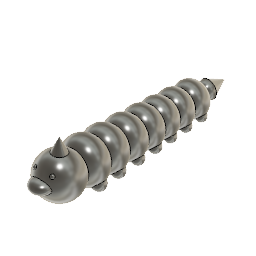
imomushi (Autodesk Fusion 360 design; units mm, degrees)
Autodesk Fusion 360 part; units mm, degrees
note: some values were not read from the file. Set by a fixed rule: which sketch regions a step uses.
sketch "スケッチ1" plane through (0, 0, 0) normal (0, 1, 0) x (1, 0, 0)
  line L0 (0, 0) -> (0, -20)
  line L1 (0, 0) -> (10, 0)
  line L2 (10, 0) -> (0, -20)
  arc A0 (10, 0) -> (0, 10) centre (0, 0) ccw
  line L3 (0, 0) -> (0, 10)
  ellipse E0 centre (0, 0) end of major axis (0, -7.5) minor radius 12.5
  line L4 (0, 7.5) -> (0, -7.5)
  line L5 (-12.5, 0) -> (12.5, 0)
  ellipse E1 centre (0, 0) end of major axis (0, -20) minor radius 25
  line L6 (0, 20) -> (0, -20)
  line L7 (-25, 0) -> (25, 0)
  circle A1 centre (0, 0) radius 7.5
  line L8 (0, -20) -> (0, 20)
  dimension "d1" = 20
  dimension "d2" = 10
  dimension "d8" = 15
  dimension "d9" = 25
  constraint coincident L0.start L1.start
  constraint vertical L0
  constraint perpendicular L0 L1
  constraint perpendicular L1 L3
  constraint perpendicular L1 L4
  constraint coincident E0 L4.start
  constraint coincident E0 L4.end
  constraint coincident E0 L5.start
  constraint coincident E0 L5.end
  constraint concentric A0 E1
  constraint parallel L0 L6
  constraint coincident E1 L6.start
  constraint coincident E1 L7.start
  constraint coincident E1 L7.end
  constraint coincident L4.end A1
  constraint parallel L6 L8
  measures "d1" distance of L0.start L0.end
  measures "d2" distance of L0.start L1.end
  measures "d8" distance of E0
revolve "回転1" add sketch "スケッチ1" angle 360 about axis through (0, 0, 1.75) along (0, 0, 1) contours L0 L1 L4 L5 L6 L7 A1 L8 | L0 L2 E0 L6 L8 | L1 L2 E0 L5 L7 A1 makes body 1
revolve "回転2" add sketch "スケッチ1" angle 360 about axis through (0, 0, 1.75) along (0, 0, 1) separate body contours L0 L1 L4 L5 L6 L7 A1 L8 | L1 L3 L4 L5 L6 L7 A1 L8 | L0 L2 E0 L6 L8 | L1 L2 E0 L5 L7 A1 | L1 A0 E0 L5 L7 A1 | A0 L3 E0 L6 L8 makes body 2
move_body "移動1" bodies 1 to x (1, 0, 0) y (0, 1, 0) z (0, 0, 1) at (0, 0, 20)
sphere "球プリミティブ1" add diameter 50 placed x (1, 0, 0) y (0, 0, -1) z (0, 1, 0) at (0, 0, 0) separate body makes body 3
sphere "球プリミティブ2" add diameter 5 placed x (1, 0, 0) y (0, 0, -1) z (0, 1, 0) at (0, 0, 0) separate body makes body 4
move_body "移動2" bodies 4 to x (1, 0, 0) y (0, 1, 0) z (0, 0, 1) at (10.0469, -18.3305, 12.2249)
mirror "ミラー1" about plane through (0, 0, 0) normal (1, 0, 0) of bodies 4 makes body 5
revolve "回転3" add sketch "スケッチ1" angle 360 about axis through (0, 0, 1.75) along (0, 0, 1) separate body contours L0 L1 L4 L5 L6 L7 A1 L8 | L1 L3 L4 L5 L6 L7 A1 L8 | L1 L2 E0 L5 L7 A1 | L1 A0 E0 L5 L7 A1 | L2 E0 L5 L7 | A0 E0 L5 L7 makes body 6
move_body "移動3" bodies 6 to x (1, 0, 0) y (0, 1, 0) z (0, 0, 1) at (0, -21.5417, 0)
revolve "回転4" add sketch "スケッチ1" angle 360 about axis through (0, 0, 1.75) along (0, 0, 1) separate body contours L0 L1 L4 L5 L6 L7 A1 L8 | L1 L3 L4 L5 L6 L7 A1 L8 | L0 L2 E0 L6 L8 | L1 L2 E0 L5 L7 A1 | L1 A0 E0 L5 L7 A1 | A0 L3 E0 L6 L8 | L2 E0 E1 L7 | L2 E0 L5 L7 | A0 E0 L5 L7 | A0 E0 E1 L6 L7 L8 makes body 7
revolve "回転5" add sketch "スケッチ1" angle 360 about axis through (0, 0, 1.75) along (0, 0, 1) separate body contours L0 L1 L4 L5 L6 L7 A1 L8 | L1 L3 L4 L5 L6 L7 A1 L8 makes body 8
move_body "移動4" bodies 8 to x (1, 0, 0) y (0, 1, 0) z (0, 0, 1) at (16.7977, -16.1117, 0)
mirror "ミラー2" about plane through (0, 0, 0) normal (1, 0, 0) of bodies 8 makes body 9
combine "結合1" operation add target body 7 tool bodies 8 9
combine "結合2" operation add target body 1 tool bodies 3 4 5 6
move_body "移動5" bodies 7 to x (1, 0, 0) y (0, 1, 0) z (0, 0, 1) at (0, 0, -35)
copy_body "ボディのコピーと貼り付け1" bodies 7 makes body 10
move_body "移動6" bodies 10 to x (1, 0, 0) y (0, 1, 0) z (0, 0, 1) at (0, 0, -20)
scale "尺度1" factor 0.95 about (0, 0, -35) bodies 10
move_body "移動7" bodies 10 to x (1, 0, 0) y (0, 1, 0) z (0, 0, 1) at (0, 0, -7)
copy_body "ボディのコピーと貼り付け2" bodies 10 makes body 11
move_body "移動8" bodies 11 to x (1, 0, 0) y (0, 1, 0) z (0, 0, 1) at (0, 0, -20)
scale "尺度2" factor 0.95 about (0, 0, -62) bodies 11
move_body "移動9" bodies 11 to x (1, 0, 0) y (0, 1, 0) z (0, 0, 1) at (0, 0, -5)
copy_body "ボディのコピーと貼り付け3" bodies 11 makes body 12
move_body "移動10" bodies 12 to x (1, 0, 0) y (0, 1, 0) z (0, 0, 1) at (0, 0, -22.5)
scale "尺度3" factor 0.95 about (0, 0, -89.5) bodies 12
copy_body "ボディのコピーと貼り付け4" bodies 12 makes body 13
move_body "移動11" bodies 13 to x (1, 0, 0) y (0, 1, 0) z (0, 0, 1) at (0, 0, -20)
scale "尺度4" factor 0.95 about (0, 0, -109.5) bodies 13
copy_body "ボディのコピーと貼り付け5" bodies 13 makes body 14
move_body "移動12" bodies 14 to x (1, 0, 0) y (0, 1, 0) z (0, 0, 1) at (0, 0, -20)
scale "尺度5" factor 0.95 about (0, 0, -129.5) bodies 14
copy_body "ボディのコピーと貼り付け6" bodies 14 makes body 15
move_body "移動13" bodies 15 to x (1, 0, 0) y (0, 1, 0) z (0, 0, 1) at (0, 0, -20)
scale "尺度6" factor 0.95 about (0, 0, -149.5) bodies 15
move_body "移動14" bodies 2 to x (1, 0, 0) y (0, -1, 0) z (0, 0, -1) at (0, 0, 0)
move_body "移動15" bodies 2 to x (1, 0, 0) y (0, 1, 0) z (0, 0, 1) at (0, 0, -188.9157)
move_body "移動16" bodies 7 to x (1, 0, 0) y (0, 1, 0) z (0, 0, 1) at (0, 0, 4)
move_body "移動17" bodies 10 11 12 13 14 15 2 to x (1, 0, 0) y (0, 1, 0) z (0, 0, 1) at (0, 0, 6)
move_body "移動18" bodies 1 to x (1, 0, 0) y (0, 0, -1) z (0, 1, 0) at (0, 0, 0)
move_body "移動19" bodies 2 to x (1, 0, 0) y (0, 1, 0) z (0, 0, 1) at (0, 0, 4)
combine "結合3" operation add target body 1 tool bodies 2 7 10 11 12 13 14 15
move_body "移動20" bodies 1 to x (1, 0, 0) y (0, 0, 1) z (0, -1, 0) at (0, 0, 0)
named bodies: "imomushi"
